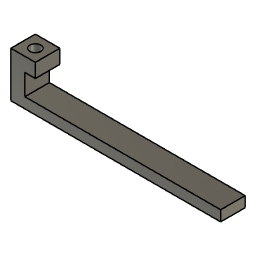
_Hook (Autodesk Fusion 360 design; units mm, degrees)
part number: 2025-05-20-09-34-36-352
Autodesk Fusion 360 part; units mm, degrees
sketch "Sketch1" plane through (0, 0, 0) normal (0, 0, 1) x (1, 0, 0)
  line L0 (0, 0) -> (76.2, 0)
  line L1 (76.2, 0) -> (76.2, 8.89)
  line L2 (76.2, 8.89) -> (0, 8.89)
  line L3 (0, 8.89) -> (0, 0)
  dimension "d1" = 76.2
  dimension "d2" = 8.89
  constraint horizontal L0
  constraint vertical L1
  constraint horizontal L2
  constraint vertical L3
  constraint coincident L0.start L3.end
  measures "d1" distance of L0.start L0.end
  measures "d2" distance of L0.start L2.end
extrude "Extrude1" add sketch "Sketch1" along normal blind 3.81
sketch "Sketch2" plane through (0, 0, 3.81) normal (0, 0, 1) x (-1, 0, 0)
  line L0 (0, -8.89) -> (0, 0)
  line L1 (0, 0) -> (-76.2, 0)
  line L2 (-76.2, 0) -> (-76.2, -8.89)
  line L3 (-76.2, -8.89) -> (0, -8.89)
  line L4 (0, 0) -> (-5.08, 0)
  line L5 (-5.08, 0) -> (-5.08, -8.89)
  line L6 (-5.08, -8.89) -> (0, -8.89)
  line L7 (0, -8.89) -> (0, 0)
  dimension "d5" = 5.08
  constraint horizontal L4
  constraint vertical L5
  constraint horizontal L6
  constraint vertical L7
  constraint coincident L0.end L1.start
  measures "d5" distance of L0.end L4.end
extrude "Extrude2" add sketch "Sketch2" along normal blind 7.62 contours L0 L1 L3 L4 L5 L6 L7
sketch "Sketch3" plane through (0, 0, 11.43) normal (0, 0, 1) x (-1, 0, 0)
  line L0 (0, -8.89) -> (0, 0)
  line L1 (0, 0) -> (-5.08, 0)
  line L2 (-5.08, 0) -> (-5.08, -8.89)
  line L3 (-5.08, -8.89) -> (0, -8.89)
  line L4 (0, 0) -> (-8.89, 0)
  line L5 (-8.89, 0) -> (-8.89, -8.89)
  line L6 (-8.89, -8.89) -> (0, -8.89)
  line L7 (0, -8.89) -> (0, 0)
  dimension "d8" = 8.89
  constraint horizontal L4
  constraint vertical L5
  constraint horizontal L6
  constraint vertical L7
  constraint coincident L0.end L1.start
  measures "d8" distance of L0.end L4.end
extrude "Extrude3" add sketch "Sketch3" along normal blind 5.08
hole "Hole1" at (4.445, 4.445, 16.51) direction (0, 0, -1) diameter 4 depth 4 tip angle 180
